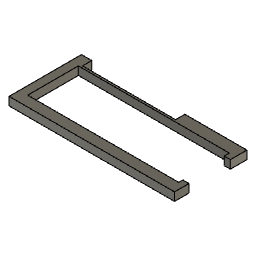
lcd bottom (Autodesk Fusion 360 design; units mm, degrees)
Autodesk Fusion 360 part; units mm, degrees
sketch "Sketch1" plane through (0, 0, 0) normal (0, 0, 1) x (1, 0, 0)
  line L0 (0, 0) -> (0, 35)
  line L1 (0, 35) -> (80, 35)
  line L2 (80, 35) -> (80, 27)
  line L3 (80, 27) -> (77, 27)
  line L4 (77, 27) -> (77, 29.5)
  line L5 (77, 29.5) -> (4, 29.5)
  line L6 (4, 29.5) -> (4, 5)
  line L7 (4, 5) -> (77, 5)
  line L8 (77, 5) -> (77, 7)
  line L9 (77, 7) -> (80, 7)
  line L10 (80, 7) -> (80, 0)
  line L11 (80, 0) -> (0, 0)
  line L12 (4.2162, 35) -> (5, 35)
  line L13 (4, 32) -> (4.2162, 32)
  line L14 (5, 35) -> (50, 35)
  line L15 (50, 35) -> (50, 30.5)
  line L16 (50, 30.5) -> (5, 30.5)
  line L17 (5, 30.5) -> (5, 35)
  dimension "d3" = 35
  dimension "d4" = 5
  dimension "d5" = 5.5
  dimension "d6" = 3
  dimension "d7" = 3
  dimension "d8" = 8
  dimension "d9" = 7
  dimension "d10" = 4
  dimension "d11" = 80
  dimension "d12" = 80
  dimension "d13" = 45
  dimension "d14" = 5
  dimension "d15" = 4.5
  constraint coincident L0.start L11.end
  constraint vertical L0
  constraint perpendicular L0 L1
  constraint perpendicular L1 L2
  constraint perpendicular L2 L3
  constraint perpendicular L1 L4
  constraint perpendicular L2 L5
  constraint perpendicular L5 L6
  constraint perpendicular L6 L7
  constraint perpendicular L7 L8
  constraint perpendicular L8 L9
  constraint perpendicular L9 L10
  constraint perpendicular L0 L11
  constraint horizontal L12
  constraint horizontal L13
  constraint coincident L1 L12.start
  constraint horizontal L14
  constraint vertical L15
  constraint horizontal L16
  constraint vertical L17
  measures "d3" distance of L0.start L0.end
  measures "d4" distance of L7 L11
  measures "d5" distance of L1 L5
  measures "d6" distance of L8 L10
  measures "d7" distance of L2 L4
  measures "d8" distance of L1 L3
  measures "d9" distance of L9 L11
  measures "d10" distance of L0 L6
  measures "d11" distance of L0 L2
  measures "d12" distance of L0 L10
  measures "d13" distance of L15.end L16.end
  measures "d14" distance of L0 L17
  measures "d15" distance of L14 L16
extrude "Extrude1" add sketch "Sketch1" along normal blind 4 contours L0 L1 L2 L3 L4 L5 L6 L7 L8 L9 L10 L11 L12 L15 L16 L17
